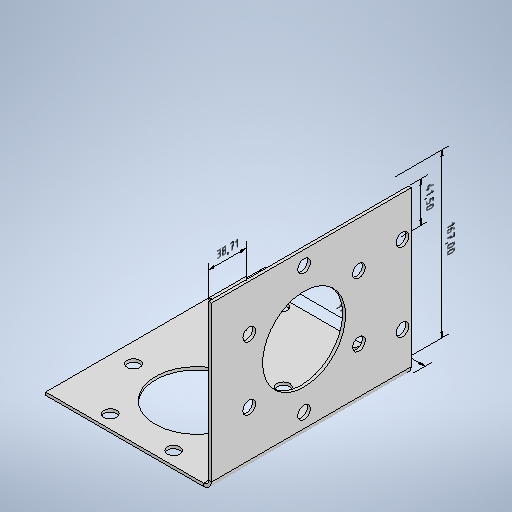
# Autodesk Inventor part: drain wall with flange
Saved by Autodesk Inventor 2025.1 (Build 291241020, 241B)
## iProperties
Created: 2024-12-09
Part Number: drain wall with flange
Material: Stainless Steel
Document SubType Name: Sheet Metal
Designer: user
Mass: 1266.46 g
Surface Area: 1122.88 cm^2
Volume: 158.308 cm^3
Density: 8 g/cm^3
Sheet Metal Rule: AISI304 3mm Die 32
Sheet Metal Width: 205.000 mm
Sheet Metal Length: 330.927 mm
Sheet Metal Area: 67840.124 mm^2
Appearance: Default
Flat Pattern Width: 20.5 cm
Flat Pattern Length: 33.0927 cm
Flat Pattern Area: 678.401 cm^2
Author: user
Autodesk Inventor part; units mm, degrees
ref_plane "YZ Plane" through (0, 0, 0) normal (1, 0, 0) x (0, 1, 0)
ref_plane "XZ Plane" through (0, 0, 0) normal (0, 1, 0) x (-1, 0, 0)
ref_plane "XY Plane" through (0, 0, 0) normal (0, 0, 1) x (1, 0, 0)
sketch "Sketch1" plane through (0, 0, 0) normal (0, 0, 1) x (1, 0, 0)
  line L0 (-85, -102.5) -> (85, -102.5)
  line L1 (85, -102.5) -> (85, 102.5)
  line L2 (85, 102.5) -> (-85, 102.5)
  line L3 (-85, 102.5) -> (-85, -102.5)
  line L4 (-85, -102.5) -> (85, 102.5) construction
  line L5 (85, -102.5) -> (-85, 102.5) construction
  circle A0 centre (0, -32.5) radius 42.5
  point P0 (0, 0)
  point P1 (0, -102.5)
  dimension "d0" = 170
  dimension "d1" = 205
  dimension "d22" = 85
  dimension "d61" = 70
  measures "d0" distance of L2.end L1.end
  measures "d1" distance of L1.end L0.end
  measures "d22" diameter of A0
  measures "d61" distance from line of L0 A0.centre
extrude "Plate1" add sketch "Sketch1" along normal blind 3
sketch "Sketch5" plane through (82, 102.5, 0) normal (1, 0, 0) x (0, 1, 0)
  line L0 (-205, 0) -> (0, 0)
  line L1 (0, 0) -> (0, 167)
  line L2 (0, 167) -> (-205, 167)
  line L3 (-205, 167) -> (-205, 0)
  constraints: 6 end point, 1 horizontal, 1 perpendicular, 1 vertical
edge flange "Flange2" height 167 angle 90 thickness 3 bend radius 5 thickness toward (1, 0, 0) relief round relief width 3 relief depth 1.5 edges at (85, 0, 3) wall of the first edge with corners at (82, -102.5, 0) (82, 102.5, 0) (82, 102.5, 167) (82, -102.5, 167)
bend "Bend2"
corner "Corner2"
sketch "Sketch6" plane through (85, -102.5, 167) normal (1, 0, 0) x (0, 0, -1)
  line L0 (159, 0) -> (159, 205) projected
  line L1 (0, 205) -> (159, 205) projected
  line L2 (0, 0) -> (0, 205) projected
  line L3 (159, 0) -> (0, 0) projected
  circle A0 centre (79.5, 95) radius 42.5
  point P0 (167, 102.5)
  point P1 (79.5, 205)
  dimension "d33" = 85
  dimension "d60" = 95
  constraints: 1 centre point, 1 midpoint, 1 vertical alignment
  measures "d33" diameter of A0
  measures "d60" distance from line of A0.centre L3
extrude "Cut1" cut sketch "Sketch6" against normal blind 3 contours A0
sketch "Sketch7" plane through (85, -102.5, 167) normal (1, 0, 0) x (0, 0, -1)
  circle A0 centre (47, 151.2917) radius 6.5
  circle A1 centre (79.5, 95) radius 42.5 projected
  circle A2 centre (79.5, 95) radius 65 construction
  line L0 (79.5, 95) -> (79.5, 137.5)
  line L1 (79.5, 95) -> (47, 151.2917)
  point P0 (167, 102.5)
  dimension "d37" = 130
  dimension "d36" = 13
  dimension "d81" = 30
  constraints: 4 end point, 1 centre point, 1 coincident, 1 vertical, 1 vertical alignment, 4 other
  measures "d36" diameter of A0
  measures "d81" angle of L0 L1
extrude "Cut2" cut sketch "Sketch7" against normal blind 3 contours A0
pattern_circular "Circular Pattern1" count 6 over 360 about axis through (85, -7.5, 87.5) along (-1, 0, 0) of "Cut2"
sketch "Sketch8" plane through (0, 0, 3) normal (0, 0, 1) x (1, 0, 0)
  circle A0 centre (-32.5, 23.7917) radius 6.5
  circle A1 centre (0, -32.5) radius 65 construction
  circle A2 centre (0, -32.5) radius 42.5 projected
  line L0 (0, 10) -> (0, -32.5)
  line L1 (0, -32.5) -> (-32.5, 23.7917)
  dimension "d44" = 130
  dimension "d43" = 13
  dimension "d82" = 30
  constraints: 4 end point, 1 centre point, 1 coincident, 1 vertical, 1 vertical alignment, 4 other
  measures "d43" diameter of A0
  measures "d82" angle of L0 L1
extrude "Cut3" cut sketch "Sketch8" against normal blind 3 contours A0
pattern_circular "Circular Pattern2" count 6 over 360 about axis through (0, -32.5, 0) along (0, 0, 1) of "Cut3"
sketch "Sketch10" plane through (85, -102.5, 167) normal (1, 0, 0) x (0, 0, -1)
  circle A0 centre (41.5, 196) radius 6.5
  circle A1 centre (121.5, 196) radius 6.5
  line L0 (159, 205) -> (0, 205) projected
  line L1 (81.5, 200.962) -> (81.5, 182.1235)
  point P0 (167, 102.5)
  dimension "d62" = 13
  dimension "d63" = 9
  dimension "d64" = 80
  dimension "d72" = 81.5
  constraints: 2 centre point, 2 end point, 1 vertical, 1 other
  measures "d62" diameter of A0
  measures "d63" distance from line of A0.centre L0
  measures "d64" distance of A1.centre A0.centre
  measures "d72" distance from line of L1 L0.end
extrude "Cut4" cut sketch "Sketch10" against normal blind 3
sketch "Sketch11" plane through (0, 0, 3) normal (0, 0, 1) x (1, 0, 0)
  circle A0 centre (-40, 93.5) radius 6.5
  circle A1 centre (40, 93.5) radius 6.5
  line L0 (0, 102.5) -> (0, 73.9677)
  line L1 (-85, 102.5) -> (77, 102.5) projected
  point P0 (0, 0)
  dimension "d67" = 13
  dimension "d68" = 80
  dimension "d69" = 9
  constraints: 2 centre point, 2 end point, 1 perpendicular, 1 point on line, 1 vertical, 1 other
  measures "d67" diameter of A0
  measures "d68" distance of A1.centre A0.centre
  measures "d69" distance from line of L1 A0.centre
extrude "Cut5" cut sketch "Sketch11" against normal blind 3
equation "\"d33\" = d22"
equation "\"d34\" = Thickness"
equation "\"d38\" = Thickness"
equation "\"d45\" = Thickness"
equation "\"d65\" = Thickness"
equation "\"d70\" = Thickness"
equation "\"d2\" = Thickness"
equation "\"d23\" = BendReliefWidth"
equation "\"d24\" = BendReliefDepth"
equation "\"d25\" = MinimumRemnant"
equation "\"d26\" = TransitionRadius"
equation "\"d29\" = BendRadius"
equation "\"d30\" = CornerReliefSize"
equation "\"d31\" = GapSize"
equation "\"d32\" = JacobiRadiusSize"
equation "\"BendReliefWidth\" = Thickness"
equation "\"BendReliefDepth\" = 0.5 * Thickness"
equation "\"CornerReliefSize\" = 4 * Thickness"
equation "\"MinimumRemnant\" = 2 * Thickness"
equation "\"TransitionRadius\" = BendRadius"
equation "\"JacobiRadiusSize\" = BendRadius"
equation "\"GapSize\" = Thickness"
equation "\"Thickness\" = 3"
equation "\"BendRadius\" = 5"
body "Solid1"
